Autodesk Fusion 360 part; units mm, degrees
(part 2 of 14)
  arc A256 (88.9, 8.89) -> (88.9, 3.81) centre (88.9, 6.35) ccw
  line L628 (88.646, 6.35) -> (89.154, 6.35)
  line L629 (88.646, 6.35) -> (89.154, 6.35)
  line L630 (88.646, 6.35) -> (89.154, 6.35)
  arc A257 (88.9, 7.62) -> (88.9, 5.08) centre (88.9, 6.35) ccw
  arc A258 (89.5414, 57.15) -> (88.2587, 57.15) centre (88.9, 57.15) ccw
  arc A259 (89.5414, 6.35) -> (88.2587, 6.35) centre (88.9, 6.35) ccw
  line L631 (88.9, 56.896) -> (88.9, 57.404)
  arc A260 (88.9, 5.08) -> (88.9, 7.62) centre (88.9, 6.35) ccw
  arc A261 (89.5414, 6.35) -> (88.2587, 6.35) centre (88.9, 6.35) ccw
  arc A262 (89.5414, 57.15) -> (88.2587, 57.15) centre (88.9, 57.15) ccw
  line L632 (88.646, 6.35) -> (89.154, 6.35)
  line L633 (88.9, 6.096) -> (88.9, 6.604)
  arc A263 (92.31, 13.414) -> (92.31, 12.906) centre (92.31, 13.16) ccw
  arc A264 (89.5414, 6.35) -> (88.2587, 6.35) centre (88.9, 6.35) ccw
  arc A265 (89.5414, 57.15) -> (88.2587, 57.15) centre (88.9, 57.15) ccw
  line L634 (88.9, 6.096) -> (88.9, 6.604)
  line L635 (88.9, 6.096) -> (88.9, 6.604)
  line L636 (88.9, 56.896) -> (88.9, 57.404)
  line L637 (88.646, 57.15) -> (89.154, 57.15)
  arc A266 (88.9, 5.08) -> (88.9, 7.62) centre (88.9, 6.35) ccw
  arc A267 (88.9, 7.62) -> (88.9, 5.08) centre (88.9, 6.35) ccw
  arc A268 (88.9, 4.7879) -> (88.9, 7.9121) centre (88.9, 6.35) ccw
  line L638 (88.9, 56.896) -> (88.9, 57.404)
  arc A269 (89.5414, 57.15) -> (88.2587, 57.15) centre (88.9, 57.15) ccw
  line L639 (88.646, 6.35) -> (89.154, 6.35)
  arc A270 (88.9, 7.9121) -> (88.9, 4.7879) centre (88.9, 6.35) ccw
  arc A271 (88.2587, 6.35) -> (89.5414, 6.35) centre (88.9, 6.35) ccw
  line L640 (88.9, 56.896) -> (88.9, 57.404)
  arc A272 (88.2587, 6.35) -> (89.5414, 6.35) centre (88.9, 6.35) ccw
  line L641 (88.646, 57.15) -> (89.154, 57.15)
  line L642 (88.646, 6.35) -> (89.154, 6.35)
  line L643 (88.646, 6.35) -> (89.154, 6.35)
  line L644 (88.9, 6.096) -> (88.9, 6.604)
  arc A273 (89.5414, 6.35) -> (88.2587, 6.35) centre (88.9, 6.35) ccw
  arc A274 (88.9, 4.7879) -> (88.9, 7.9121) centre (88.9, 6.35) ccw
  arc A275 (88.9, 7.9121) -> (88.9, 4.7879) centre (88.9, 6.35) ccw
  line L645 (88.646, 6.35) -> (89.154, 6.35)
  arc A276 (87.3252, 6.35) -> (90.4748, 6.35) centre (88.9, 6.35) ccw
  arc A277 (87.3252, 6.35) -> (90.4748, 6.35) centre (88.9, 6.35) ccw
  arc A278 (89.5414, 6.35) -> (88.2587, 6.35) centre (88.9, 6.35) ccw
  arc A279 (89.5414, 6.35) -> (88.2587, 6.35) centre (88.9, 6.35) ccw
  arc A280 (88.9, 3.81) -> (88.9, 8.89) centre (88.9, 6.35) ccw
  arc A281 (92.31, 13.668) -> (92.31, 12.652) centre (92.31, 13.16) ccw
  arc A282 (88.9, 8.89) -> (88.9, 3.81) centre (88.9, 6.35) ccw
  arc A283 (90.4748, 57.15) -> (87.3252, 57.15) centre (88.9, 57.15) ccw
  arc A284 (88.2587, 57.15) -> (89.5414, 57.15) centre (88.9, 57.15) ccw
  line L646 (88.9, 6.096) -> (88.9, 6.604)
  arc A285 (92.31, 12.906) -> (92.31, 13.414) centre (92.31, 13.16) ccw
  arc A286 (88.2587, 6.35) -> (89.5414, 6.35) centre (88.9, 6.35) ccw
  arc A287 (88.9, 8.89) -> (88.9, 3.81) centre (88.9, 6.35) ccw
  arc A288 (90.4748, 6.35) -> (87.3252, 6.35) centre (88.9, 6.35) ccw
  line L647 (88.646, 6.35) -> (89.154, 6.35)
  arc A289 (88.2587, 6.35) -> (89.5414, 6.35) centre (88.9, 6.35) ccw
  line L648 (88.9, 6.096) -> (88.9, 6.604)
  arc A290 (89.5414, 6.35) -> (88.2587, 6.35) centre (88.9, 6.35) ccw
  arc A291 (88.2587, 6.35) -> (89.5414, 6.35) centre (88.9, 6.35) ccw
  arc A292 (88.2587, 57.15) -> (89.5414, 57.15) centre (88.9, 57.15) ccw
  arc A293 (88.9, 58.42) -> (88.9, 55.88) centre (88.9, 57.15) ccw
  line L649 (6.35, 56.896) -> (6.35, 57.404)
  arc A294 (88.9, 58.42) -> (88.9, 55.88) centre (88.9, 57.15) ccw
  arc A295 (6.9913, 57.15) -> (5.7086, 57.15) centre (6.35, 57.15) ccw
  arc A296 (4.7752, 57.15) -> (7.9248, 57.15) centre (6.35, 57.15) ccw
  arc A297 (89.5414, 57.15) -> (88.2587, 57.15) centre (88.9, 57.15) ccw
  line L650 (88.646, 57.15) -> (89.154, 57.15)
  arc A298 (88.9, 5.08) -> (88.9, 7.62) centre (88.9, 6.35) ccw
  arc A299 (88.9, 7.62) -> (88.9, 5.08) centre (88.9, 6.35) ccw
  arc A300 (89.5414, 57.15) -> (88.2587, 57.15) centre (88.9, 57.15) ccw
  arc A301 (88.2587, 57.15) -> (89.5414, 57.15) centre (88.9, 57.15) ccw
  arc A302 (88.9, 6.0007) -> (88.9, 6.6992) centre (88.9, 6.35) ccw
  arc A303 (89.5414, 57.15) -> (88.2587, 57.15) centre (88.9, 57.15) ccw
  line L651 (88.646, 57.15) -> (89.154, 57.15)
  arc A304 (88.9, 54.61) -> (88.9, 59.69) centre (88.9, 57.15) ccw
  arc A305 (88.9, 57.931) -> (88.9, 56.3689) centre (88.9, 57.15) ccw
  arc A306 (6.9913, 57.15) -> (5.7086, 57.15) centre (6.35, 57.15) ccw
  arc A307 (88.9, 54.61) -> (88.9, 59.69) centre (88.9, 57.15) ccw
  arc A308 (88.9, 58.42) -> (88.9, 55.88) centre (88.9, 57.15) ccw
  arc A309 (88.9, 58.7121) -> (88.9, 55.5879) centre (88.9, 57.15) ccw
  arc A310 (5.7086, 57.15) -> (6.9913, 57.15) centre (6.35, 57.15) ccw
  line L652 (88.646, 57.15) -> (89.154, 57.15)
  arc A311 (89.5414, 57.15) -> (88.2587, 57.15) centre (88.9, 57.15) ccw
  arc A312 (88.9, 57.4992) -> (88.9, 56.8007) centre (88.9, 57.15) ccw
  line L653 (6.096, 57.15) -> (6.604, 57.15)
  arc A313 (88.2587, 57.15) -> (89.5414, 57.15) centre (88.9, 57.15) ccw
  arc A314 (5.7086, 57.15) -> (6.9913, 57.15) centre (6.35, 57.15) ccw
  line L654 (6.096, 57.15) -> (6.604, 57.15)
  arc A315 (90.4748, 57.15) -> (87.3252, 57.15) centre (88.9, 57.15) ccw
  arc A316 (88.9, 6.6992) -> (88.9, 6.0007) centre (88.9, 6.35) ccw
  line L655 (88.9, 56.896) -> (88.9, 57.404)
  arc A317 (88.2587, 57.15) -> (89.5414, 57.15) centre (88.9, 57.15) ccw
  arc A318 (88.9, 5.08) -> (88.9, 7.62) centre (88.9, 6.35) ccw
  arc A319 (88.2587, 57.15) -> (89.5414, 57.15) centre (88.9, 57.15) ccw
  line L656 (88.646, 57.15) -> (89.154, 57.15)
  line L657 (88.9, 56.896) -> (88.9, 57.404)
  arc A320 (87.3252, 57.15) -> (90.4748, 57.15) centre (88.9, 57.15) ccw
  arc A321 (89.5414, 57.15) -> (88.2587, 57.15) centre (88.9, 57.15) ccw
  line L658 (88.646, 57.15) -> (89.154, 57.15)
  line L659 (88.9, 56.896) -> (88.9, 57.404)
  arc A322 (88.9, 7.62) -> (88.9, 5.08) centre (88.9, 6.35) ccw
  arc A323 (87.3252, 57.15) -> (90.4748, 57.15) centre (88.9, 57.15) ccw
  arc A324 (88.2587, 57.15) -> (89.5414, 57.15) centre (88.9, 57.15) ccw
  arc A325 (88.9, 8.89) -> (88.9, 3.81) centre (88.9, 6.35) ccw
  arc A326 (88.9, 59.69) -> (88.9, 54.61) centre (88.9, 57.15) ccw
  line L660 (88.646, 57.15) -> (89.154, 57.15)
  line L661 (88.9, 56.896) -> (88.9, 57.404)
  arc A327 (88.9, 3.81) -> (88.9, 8.89) centre (88.9, 6.35) ccw
  line L662 (88.646, 57.15) -> (89.154, 57.15)
  arc A328 (88.2587, 57.15) -> (89.5414, 57.15) centre (88.9, 57.15) ccw
  arc A329 (6.9913, 57.15) -> (5.7086, 57.15) centre (6.35, 57.15) ccw
  arc A330 (6.9913, 57.15) -> (5.7086, 57.15) centre (6.35, 57.15) ccw
  arc A331 (88.9, 59.69) -> (88.9, 54.61) centre (88.9, 57.15) ccw
  arc A332 (88.9, 58.7121) -> (88.9, 55.5879) centre (88.9, 57.15) ccw
  arc A333 (88.9, 58.42) -> (88.9, 55.88) centre (88.9, 57.15) ccw
  arc A334 (88.9, 55.88) -> (88.9, 58.42) centre (88.9, 57.15) ccw
  arc A335 (88.9, 55.88) -> (88.9, 58.42) centre (88.9, 57.15) ccw
  arc A336 (4.7752, 57.15) -> (7.9248, 57.15) centre (6.35, 57.15) ccw
  arc A337 (88.9, 55.88) -> (88.9, 58.42) centre (88.9, 57.15) ccw
  line L663 (6.35, 56.896) -> (6.35, 57.404)
  line L664 (21.5392, 25.527) -> (22.1488, 25.527)
  arc A338 (23.16, 24.4688) -> (23.16, 24.4692) centre (23.16, 24.469) ccw
  arc A339 (21.544, 25.5688) -> (21.544, 25.5692) centre (21.544, 25.569) ccw
  line L665 (23.16, 25.569) -> (22.56, 25.569)
  arc A340 (22.144, 25.5688) -> (22.144, 25.5692) centre (22.144, 25.569) ccw
  line L666 (22.5552, 24.894) -> (23.1648, 24.894)
  line L667 (21.5392, 24.511) -> (21.5392, 25.527)
  arc A341 (22.56, 25.5688) -> (22.56, 25.5692) centre (22.56, 25.569) ccw
  line L668 (22.1488, 25.527) -> (22.1488, 24.511)
  line L669 (68.836, 31.9532) -> (69.086, 31.9532)
  line L670 (69.469, 32.5628) -> (69.469, 31.9532)
  arc A342 (21.544, 24.4688) -> (21.544, 24.4692) centre (21.544, 24.469) ccw
  line L671 (22.1488, 25.144) -> (21.5392, 25.144)
  line L672 (68.453, 31.9532) -> (68.453, 32.5628)
  line L673 (22.144, 24.469) -> (22.144, 25.569)
  line L674 (22.56, 24.469) -> (23.16, 24.469)
  arc A343 (23.16, 25.5688) -> (23.16, 25.5692) centre (23.16, 25.569) ccw
  arc A344 (22.56, 25.5692) -> (22.56, 25.5688) centre (22.56, 25.569) ccw
  line L675 (22.56, 25.569) -> (22.56, 24.469)
  line L676 (68.453, 32.5628) -> (69.469, 32.5628)
  line L677 (69.469, 32.5628) -> (69.469, 31.9532)
  line L678 (68.453, 31.9532) -> (68.453, 32.5628)
  arc A345 (21.544, 24.4692) -> (21.544, 24.4688) centre (21.544, 24.469) ccw
  line L679 (21.5392, 25.144) -> (21.5392, 24.894)
  arc A346 (23.16, 24.4692) -> (23.16, 24.4688) centre (23.16, 24.469) ccw
  arc A347 (22.144, 25.5692) -> (22.144, 25.5688) centre (22.144, 25.569) ccw
  line L680 (4.3028, 23.1572) -> (4.9124, 23.1572)
  arc A348 (4.9076, 22.0989) -> (4.9076, 22.0994) centre (4.9076, 22.0992) ccw
  line L681 (23.1648, 25.527) -> (23.1648, 24.511)
  line L682 (4.3076, 22.0992) -> (4.9076, 22.0992)
  line L683 (4.9124, 23.1572) -> (4.9124, 22.1412)
  line L684 (23.1648, 24.511) -> (22.5552, 24.511)
  line L685 (23.1648, 24.511) -> (22.5552, 24.511)
  line L686 (4.3028, 22.5242) -> (4.9124, 22.5242)
  line L687 (4.9076, 23.1992) -> (4.3076, 23.1992)
  line L688 (16.4412, 14.992) -> (15.0188, 14.992)
  arc A349 (4.3076, 23.1989) -> (4.3076, 23.1994) centre (4.3076, 23.1992) ccw
  line L689 (69.469, 31.9532) -> (68.453, 31.9532)
  line L690 (15.0188, 12.706) -> (16.4412, 12.706)
  line L691 (4.3028, 22.1412) -> (4.3028, 23.1572)
  line L692 (22.5552, 25.144) -> (22.5552, 24.894)
  line L693 (68.453, 32.5628) -> (69.469, 32.5628)
  arc A350 (4.9076, 22.0994) -> (4.9076, 22.0989) centre (4.9076, 22.0992) ccw
  line L694 (4.9124, 22.1412) -> (4.3028, 22.1412)
  line L695 (23.1648, 25.527) -> (23.1648, 24.511)
  line L696 (22.5552, 25.527) -> (23.1648, 25.527)
  line L697 (23.1648, 25.144) -> (22.5552, 25.144)
  line L698 (22.5552, 25.527) -> (23.1648, 25.527)
  line L699 (4.3028, 22.7741) -> (4.3028, 22.5242)
  line L700 (4.3028, 22.1412) -> (4.3028, 23.1572)
  arc A351 (16.455, 12.7488) -> (16.455, 12.7493) centre (16.455, 12.749) ccw
  line L701 (16.455, 14.949) -> (15.005, 14.949)
  line L702 (22.5552, 24.511) -> (22.5552, 25.527)
  arc A352 (16.455, 12.7493) -> (16.455, 12.7488) centre (16.455, 12.749) ccw
  line L703 (23.1648, 24.894) -> (23.1648, 25.144)
  line L704 (4.3076, 23.1992) -> (4.3076, 22.0992)
  line L705 (16.455, 12.749) -> (16.455, 14.949)
  line L706 (4.9124, 22.1412) -> (4.3028, 22.1412)
  line L707 (22.5552, 24.511) -> (22.5552, 25.527)
  line L708 (4.9124, 22.5242) -> (4.9124, 22.7741)
  line L709 (4.9124, 22.7741) -> (4.3028, 22.7741)
  arc A353 (4.3076, 22.0989) -> (4.3076, 22.0994) centre (4.3076, 22.0992) ccw
  line L710 (68.58, 22.35) -> (68.58, 22.7)
  line L711 (68.58, 22.35) -> (68.58, 22.7)
  line L712 (4.9076, 22.0992) -> (4.9076, 23.1992)
  line L713 (16.4412, 12.706) -> (16.4412, 14.992)
  line L714 (68.745, 22.54) -> (68.415, 22.54)
  arc A354 (4.3076, 23.1994) -> (4.3076, 23.1989) centre (4.3076, 23.1992) ccw
  line L715 (16.405, 14.699) -> (15.055, 14.699)
  arc A355 (15.005, 14.9492) -> (15.005, 14.9488) centre (15.005, 14.949) ccw
  arc A356 (4.3076, 22.0994) -> (4.3076, 22.0989) centre (4.3076, 22.0992) ccw
  line L716 (16.405, 14.699) -> (15.055, 14.699)
  arc A357 (15.005, 14.9488) -> (15.005, 14.9492) centre (15.005, 14.949) ccw
  arc A358 (4.9076, 23.1994) -> (4.9076, 23.1989) centre (4.9076, 23.1992) ccw
  line L717 (16.4412, 14.992) -> (15.0188, 14.992)
  line L718 (15.0188, 12.706) -> (16.4412, 12.706)
  line L719 (68.58, 22.35) -> (68.58, 22.7)
  arc A359 (82.781, 27.1767) -> (82.781, 27.1132) centre (82.781, 27.145) ccw
  arc A360 (83.081, 27.1767) -> (83.081, 27.1132) centre (83.081, 27.145) ccw
  line L720 (68.7578, 22.5552) -> (68.4022, 22.5552)
  line L721 (15.0188, 14.992) -> (15.0188, 12.706)
  arc A361 (16.455, 14.9492) -> (16.455, 14.9488) centre (16.455, 14.949) ccw
  arc A362 (16.455, 14.9488) -> (16.455, 14.9492) centre (16.455, 14.949) ccw
  arc A363 (4.9076, 23.1989) -> (4.9076, 23.1994) centre (4.9076, 23.1992) ccw
  line L722 (15.0188, 14.992) -> (15.0188, 12.706)
  line L723 (15.005, 14.949) -> (15.005, 12.749)
  line L724 (15.005, 12.749) -> (16.455, 12.749)
  line L725 (16.4412, 12.706) -> (16.4412, 14.992)
  line L726 (16.405, 12.999) -> (15.055, 12.999)
  line L727 (4.3028, 23.1572) -> (4.9124, 23.1572)
  line L728 (68.43, 21.75) -> (68.73, 21.75)
  line L729 (68.73, 21.75) -> (68.73, 22.7)
  line L730 (4.9124, 23.1572) -> (4.9124, 22.1412)
  arc A364 (68.43, 22.7317) -> (68.43, 22.6682) centre (68.43, 22.7) ccw
  arc A365 (33.1967, 60.17) -> (33.1972, 60.17) centre (33.197, 60.17) ccw
  arc A366 (33.1967, 58.138) -> (33.1972, 58.138) centre (33.197, 58.138) ccw
  arc A367 (34.2972, 60.17) -> (34.2967, 60.17) centre (34.297, 60.17) ccw
  line L731 (33.872, 58.7428) -> (33.622, 58.7428)
  line L732 (33.622, 58.1332) -> (33.872, 58.1332)
  line L733 (33.622, 58.438) -> (33.072, 58.438)
  arc A368 (34.2967, 58.138) -> (34.2972, 58.138) centre (34.297, 58.138) ccw
  line L734 (34.422, 58.438) -> (33.872, 58.438)
  line L735 (33.239, 58.1332) -> (33.239, 58.7428)
  arc A369 (34.2967, 59.754) -> (34.2972, 59.754) centre (34.297, 59.754) ccw
  line L736 (33.872, 60.7748) -> (33.622, 60.7748)
  line L737 (34.255, 60.1652) -> (33.239, 60.1652)
  line L738 (33.239, 58.7428) -> (34.255, 58.7428)
  line L739 (34.422, 58.438) -> (33.872, 58.438)
  line L740 (34.255, 60.7748) -> (34.255, 60.1652)
  line L741 (33.622, 60.7748) -> (33.622, 60.1652)
  line L742 (34.255, 59.7588) -> (34.255, 59.1492)
  line L743 (34.255, 59.1492) -> (33.239, 59.1492)
  line L744 (34.255, 58.7428) -> (34.255, 58.1332)
  line L745 (33.239, 59.1492) -> (33.239, 59.7588)
  arc A370 (34.2967, 59.154) -> (34.2972, 59.154) centre (34.297, 59.154) ccw
  arc A371 (34.2972, 60.77) -> (34.2967, 60.77) centre (34.297, 60.77) ccw
  line L746 (33.239, 59.7588) -> (34.255, 59.7588)
  line L747 (33.622, 60.1652) -> (33.872, 60.1652)
  line L748 (34.255, 59.1492) -> (33.239, 59.1492)
  arc A372 (33.1967, 59.154) -> (33.1972, 59.154) centre (33.197, 59.154) ccw
  arc A373 (34.2967, 60.77) -> (34.2972, 60.77) centre (34.297, 60.77) ccw
  arc A374 (33.1972, 59.154) -> (33.1967, 59.154) centre (33.197, 59.154) ccw
  line L749 (33.239, 60.7748) -> (34.255, 60.7748)
  arc A375 (33.1972, 59.754) -> (33.1967, 59.754) centre (33.197, 59.754) ccw
  line L750 (33.239, 59.7588) -> (34.255, 59.7588)
  line L751 (34.255, 60.1652) -> (33.239, 60.1652)
  line L752 (34.422, 59.454) -> (33.872, 59.454)
  line L753 (33.622, 59.7588) -> (33.622, 59.1492)
  line L754 (34.422, 59.454) -> (33.872, 59.454)
  line L755 (34.255, 59.7588) -> (34.255, 59.1492)
  arc A376 (33.1967, 59.754) -> (33.1972, 59.754) centre (33.197, 59.754) ccw
  line L756 (33.872, 59.7588) -> (33.622, 59.7588)
  arc A377 (34.2972, 59.154) -> (34.2967, 59.154) centre (34.297, 59.154) ccw
  line L757 (33.622, 59.454) -> (33.072, 59.454)
  line L758 (34.297, 60.17) -> (34.297, 60.77)
  line L759 (33.622, 59.454) -> (33.072, 59.454)
  arc A378 (34.2972, 59.754) -> (34.2967, 59.754) centre (34.297, 59.754) ccw
  line L760 (33.197, 60.17) -> (34.297, 60.17)
  line L761 (33.239, 60.1652) -> (33.239, 60.7748)
  arc A379 (33.1972, 60.77) -> (33.1967, 60.77) centre (33.197, 60.77) ccw
  line L762 (33.872, 60.1652) -> (33.872, 60.7748)
  arc A380 (34.2967, 60.17) -> (34.2972, 60.17) centre (34.297, 60.17) ccw
  line L763 (34.255, 60.7748) -> (34.255, 60.1652)
  line L764 (34.297, 60.77) -> (33.197, 60.77)
  line L765 (34.422, 59.454) -> (33.872, 59.454)
  line L766 (33.239, 60.1652) -> (33.239, 60.7748)
  line L767 (33.197, 60.77) -> (33.197, 60.17)
  line L768 (33.239, 60.7748) -> (34.255, 60.7748)
  arc A381 (33.1972, 60.17) -> (33.1967, 60.17) centre (33.197, 60.17) ccw
  line L769 (33.239, 59.1492) -> (33.239, 59.7588)
  line L770 (33.622, 59.1492) -> (33.872, 59.1492)
  arc A382 (33.1967, 60.77) -> (33.1972, 60.77) centre (33.197, 60.77) ccw
  line L771 (33.239, 61.7908) -> (34.255, 61.7908)
  arc A383 (34.2967, 61.186) -> (34.2972, 61.186) centre (34.297, 61.186) ccw
  line L772 (34.422, 61.486) -> (33.872, 61.486)
  line L773 (33.197, 61.186) -> (34.297, 61.186)
  line L774 (34.255, 61.1812) -> (33.239, 61.1812)
  line L775 (33.622, 59.454) -> (33.072, 59.454)
  line L776 (33.872, 61.1812) -> (33.872, 61.7908)
  line L777 (33.622, 61.1812) -> (33.872, 61.1812)
  line L778 (33.622, 60.47) -> (33.072, 60.47)
  arc A384 (34.2967, 61.786) -> (34.2972, 61.786) centre (34.297, 61.786) ccw
  line L779 (33.622, 60.47) -> (33.072, 60.47)
  line L780 (34.422, 61.486) -> (33.872, 61.486)
  line L781 (34.422, 60.47) -> (33.872, 60.47)
  line L782 (33.239, 61.1812) -> (33.239, 61.7908)
  line L783 (34.297, 61.186) -> (34.297, 61.786)
  arc A385 (33.1967, 61.786) -> (33.1972, 61.786) centre (33.197, 61.786) ccw
  line L784 (33.622, 61.7908) -> (33.622, 61.1812)
  line L785 (34.255, 61.7908) -> (34.255, 61.1812)
  line L786 (34.297, 61.786) -> (33.197, 61.786)
  arc A386 (33.1972, 61.186) -> (33.1967, 61.186) centre (33.197, 61.186) ccw
  arc A387 (33.1972, 61.786) -> (33.1967, 61.786) centre (33.197, 61.786) ccw
  line L787 (34.422, 60.47) -> (33.872, 60.47)
  line L788 (34.255, 61.1812) -> (33.239, 61.1812)
  line L789 (34.255, 61.7908) -> (34.255, 61.1812)
  line L790 (33.197, 61.786) -> (33.197, 61.186)
  line L791 (33.239, 61.1812) -> (33.239, 61.7908)
  arc A388 (33.1967, 61.186) -> (33.1972, 61.186) centre (33.197, 61.186) ccw
  arc A389 (34.2972, 61.786) -> (34.2967, 61.786) centre (34.297, 61.786) ccw
  line L792 (34.422, 60.47) -> (33.872, 60.47)
  line L793 (30.311, 59.228) -> (30.311, 58.628)
  line L794 (30.736, 58.6232) -> (30.986, 58.6232)
  line L795 (33.622, 61.486) -> (33.072, 61.486)
  line L796 (33.622, 60.47) -> (33.072, 60.47)
  arc A390 (34.2972, 61.186) -> (34.2967, 61.186) centre (34.297, 61.186) ccw
  line L797 (30.311, 58.628) -> (31.411, 58.628)
  line L798 (33.872, 61.7908) -> (33.622, 61.7908)
  arc A391 (31.4112, 58.628) -> (31.4108, 58.628) centre (31.411, 58.628) ccw
  line L799 (33.622, 61.486) -> (33.072, 61.486)
  line L800 (30.353, 58.6232) -> (30.353, 59.2328)
  line L801 (33.622, 61.486) -> (33.072, 61.486)
  line L802 (33.239, 61.7908) -> (34.255, 61.7908)
  line L803 (31.411, 59.228) -> (30.311, 59.228)
  line L804 (30.311, 57.612) -> (31.411, 57.612)
  line L805 (34.422, 61.486) -> (33.872, 61.486)
  line L806 (31.411, 57.612) -> (31.411, 58.212)
  line L807 (31.411, 58.212) -> (30.311, 58.212)
  line L808 (31.369, 59.2328) -> (31.369, 58.6232)
  line L809 (30.986, 58.928) -> (31.536, 58.928)
  line L810 (30.311, 58.212) -> (30.311, 57.612)
  arc A392 (31.4108, 59.228) -> (31.4112, 59.228) centre (31.411, 59.228) ccw
  arc A393 (31.4112, 57.612) -> (31.4108, 57.612) centre (31.411, 57.612) ccw
  line L811 (30.186, 58.928) -> (30.736, 58.928)
  line L812 (30.186, 58.928) -> (30.736, 58.928)
  line L813 (30.353, 58.2168) -> (31.369, 58.2168)
  line L814 (30.353, 59.2328) -> (31.369, 59.2328)
  arc A394 (31.4108, 57.612) -> (31.4112, 57.612) centre (31.411, 57.612) ccw
  arc A395 (31.4108, 58.212) -> (31.4112, 58.212) centre (31.411, 58.212) ccw
  arc A396 (30.3112, 59.228) -> (30.3108, 59.228) centre (30.311, 59.228) ccw
  line L815 (31.369, 58.6232) -> (30.353, 58.6232)
  arc A397 (30.3112, 57.612) -> (30.3108, 57.612) centre (30.311, 57.612) ccw
  line L816 (31.369, 57.6072) -> (30.353, 57.6072)
  line L817 (30.353, 57.6072) -> (30.353, 58.2168)
  line L818 (30.736, 59.2328) -> (30.736, 58.6232)
  arc A398 (31.4108, 58.628) -> (31.4112, 58.628) centre (31.411, 58.628) ccw
  line L819 (30.186, 58.928) -> (30.736, 58.928)
  line L820 (30.353, 58.6232) -> (30.353, 59.2328)
  arc A399 (30.3112, 58.628) -> (30.3108, 58.628) centre (30.311, 58.628) ccw
  arc A400 (30.3108, 57.612) -> (30.3112, 57.612) centre (30.311, 57.612) ccw
  line L821 (30.986, 58.928) -> (31.536, 58.928)
  line L822 (31.369, 58.2168) -> (31.369, 57.6072)
  arc A401 (30.3108, 58.628) -> (30.3112, 58.628) centre (30.311, 58.628) ccw
  line L823 (31.369, 58.6232) -> (30.353, 58.6232)
  arc A402 (31.4112, 58.212) -> (31.4108, 58.212) centre (31.411, 58.212) ccw
  arc A403 (30.3108, 58.212) -> (30.3112, 58.212) centre (30.311, 58.212) ccw
  arc A404 (30.3112, 58.212) -> (30.3108, 58.212) centre (30.311, 58.212) ccw
  line L824 (30.736, 58.2168) -> (30.736, 57.6072)
  arc A405 (31.4112, 59.228) -> (31.4108, 59.228) centre (31.411, 59.228) ccw
  line L825 (31.411, 58.628) -> (31.411, 59.228)
  line L826 (31.369, 59.2328) -> (31.369, 58.6232)
  line L827 (30.986, 59.2328) -> (30.736, 59.2328)
  line L828 (30.986, 58.6232) -> (30.986, 59.2328)
  line L829 (29.7688, 50.165) -> (29.1592, 50.165)
  line L830 (30.186, 57.912) -> (30.736, 57.912)
  line L831 (30.186, 57.912) -> (30.736, 57.912)
  line L832 (30.986, 57.6072) -> (30.986, 58.2168)
  line L833 (29.464, 51.348) -> (29.464, 50.798)
  arc A406 (29.164, 51.2232) -> (29.164, 51.2228) centre (29.164, 51.223) ccw
  line L834 (29.7688, 51.181) -> (29.7688, 50.165)
  line L835 (29.164, 50.123) -> (29.764, 50.123)
  line L836 (30.986, 57.912) -> (31.536, 57.912)
  arc A407 (29.764, 50.1232) -> (29.764, 50.1228) centre (29.764, 50.123) ccw
  arc A408 (29.164, 50.1232) -> (29.164, 50.1228) centre (29.164, 50.123) ccw
  line L837 (30.986, 57.912) -> (31.536, 57.912)
  line L838 (29.1592, 50.548) -> (29.7688, 50.548)
  arc A409 (29.764, 51.2228) -> (29.764, 51.2232) centre (29.764, 51.223) ccw
  line L839 (30.986, 58.928) -> (31.536, 58.928)
  line L840 (29.1592, 50.798) -> (29.1592, 50.548)
  line L841 (29.1592, 51.181) -> (29.7688, 51.181)
  arc A410 (30.3108, 59.228) -> (30.3112, 59.228) centre (30.311, 59.228) ccw
  line L842 (31.369, 58.2168) -> (31.369, 57.6072)
  line L843 (31.369, 57.6072) -> (30.353, 57.6072)
  line L844 (30.986, 57.912) -> (31.536, 57.912)
  arc A411 (29.164, 50.1228) -> (29.164, 50.1232) centre (29.164, 50.123) ccw
  line L845 (30.353, 57.6072) -> (30.353, 58.2168)
  line L846 (29.7688, 51.181) -> (29.7688, 50.165)
  line L847 (29.164, 51.223) -> (29.164, 50.123)
  arc A412 (29.764, 50.1228) -> (29.764, 50.1232) centre (29.764, 50.123) ccw
  line L848 (29.464, 51.348) -> (29.464, 50.798)
  line L849 (29.764, 51.223) -> (29.164, 51.223)
  arc A413 (29.164, 51.2228) -> (29.164, 51.2232) centre (29.164, 51.223) ccw
  line L850 (30.353, 59.2328) -> (31.369, 59.2328)
  line L851 (30.186, 57.912) -> (30.736, 57.912)
  line L852 (29.1592, 50.165) -> (29.1592, 51.181)
  line L853 (29.1592, 50.165) -> (29.1592, 51.181)
  line L854 (29.7688, 50.548) -> (29.7688, 50.798)
  arc A414 (29.764, 51.2232) -> (29.764, 51.2228) centre (29.764, 51.223) ccw
  line L855 (29.1592, 51.181) -> (29.7688, 51.181)
  line L856 (30.736, 57.6072) -> (30.986, 57.6072)
  line L857 (29.7688, 50.798) -> (29.1592, 50.798)
  line L858 (29.7688, 50.165) -> (29.1592, 50.165)
  line L859 (29.464, 51.348) -> (29.464, 50.798)
  line L860 (30.353, 58.2168) -> (31.369, 58.2168)
  line L861 (29.764, 50.123) -> (29.764, 51.223)
  arc A415 (75.357, 33.3588) -> (75.357, 33.3592) centre (75.357, 33.359) ccw
  line L862 (75.3618, 34.034) -> (74.7522, 34.034)
  line L863 (75.3618, 33.401) -> (74.7522, 33.401)
  line L864 (30.986, 58.2168) -> (30.736, 58.2168)
  line L865 (75.357, 33.359) -> (75.357, 34.459)
  line L866 (75.357, 34.459) -> (74.757, 34.459)
  line L867 (74.7522, 33.401) -> (74.7522, 34.417)
  arc A416 (74.757, 34.4592) -> (74.757, 34.4588) centre (74.757, 34.459) ccw
  arc A417 (74.757, 33.3588) -> (74.757, 33.3592) centre (74.757, 33.359) ccw
  line L868 (74.7522, 34.417) -> (75.3618, 34.417)
  line L869 (75.3618, 34.417) -> (75.3618, 33.401)
  arc A418 (77.043, 54.9058) -> (77.043, 54.9062) centre (77.043, 54.906) ccw
  line L870 (75.057, 34.034) -> (75.057, 34.584)
  arc A419 (74.757, 34.4588) -> (74.757, 34.4592) centre (74.757, 34.459) ccw
  line L871 (75.3618, 33.784) -> (75.3618, 34.034)
  line L872 (77.043, 53.806) -> (77.643, 53.806)
  arc A420 (77.643, 53.8058) -> (77.643, 53.8062) centre (77.643, 53.806) ccw
  line L873 (77.043, 54.906) -> (77.043, 53.806)
  line L874 (29.464, 50.548) -> (29.464, 49.998)
  arc A421 (77.643, 53.8062) -> (77.643, 53.8058) centre (77.643, 53.806) ccw
  arc A422 (77.643, 54.9058) -> (77.643, 54.9062) centre (77.643, 54.906) ccw
  arc A423 (75.357, 34.4592) -> (75.357, 34.4588) centre (75.357, 34.459) ccw
  line L875 (77.0382, 54.231) -> (77.6478, 54.231)
  arc A424 (74.757, 33.3592) -> (74.757, 33.3588) centre (74.757, 33.359) ccw
  arc A425 (77.643, 54.9062) -> (77.643, 54.9058) centre (77.643, 54.906) ccw
  line L876 (74.757, 33.359) -> (75.357, 33.359)
  line L877 (77.643, 54.906) -> (77.043, 54.906)
  line L878 (75.057, 33.234) -> (75.057, 33.784)
  line L879 (74.757, 34.459) -> (74.757, 33.359)
  line L880 (74.7522, 34.417) -> (75.3618, 34.417)
  line L881 (75.3618, 34.417) -> (75.3618, 33.401)
  line L882 (75.057, 33.234) -> (75.057, 33.784)
  line L883 (34.802, 40.8552) -> (34.802, 41.4648)
  arc A426 (34.7602, 40.86) -> (34.7598, 40.86) centre (34.76, 40.86) ccw
  arc A427 (35.8597, 41.46) -> (35.8602, 41.46) centre (35.86, 41.46) ccw
  line L884 (29.464, 50.548) -> (29.464, 49.998)
  arc A428 (77.043, 53.8062) -> (77.043, 53.8058) centre (77.043, 53.806) ccw
  line L885 (34.76, 40.86) -> (35.86, 40.86)
  line L886 (77.643, 53.806) -> (77.643, 54.906)
  line L887 (75.057, 34.034) -> (75.057, 34.584)
  line L888 (77.0382, 53.848) -> (77.0382, 54.864)
  line L889 (74.7522, 34.034) -> (74.7522, 33.784)
  line L890 (77.6478, 53.848) -> (77.0382, 53.848)
  line L891 (77.6478, 54.231) -> (77.6478, 54.481)
  arc A429 (77.043, 53.8058) -> (77.043, 53.8062) centre (77.043, 53.806) ccw
  arc A430 (34.7598, 41.46) -> (34.7602, 41.46) centre (34.76, 41.46) ccw
  arc A431 (35.8602, 41.46) -> (35.8597, 41.46) centre (35.86, 41.46) ccw
  arc A432 (75.357, 33.3592) -> (75.357, 33.3588) centre (75.357, 33.359) ccw
  line L892 (75.3618, 33.401) -> (74.7522, 33.401)
  line L893 (74.7522, 33.401) -> (74.7522, 34.417)
  arc A433 (75.357, 34.4588) -> (75.357, 34.4592) centre (75.357, 34.459) ccw
  line L894 (77.0382, 54.864) -> (77.6478, 54.864)
  line L895 (77.0382, 54.481) -> (77.0382, 54.231)
  line L896 (74.7522, 33.784) -> (75.3618, 33.784)
  line L897 (75.057, 33.234) -> (75.057, 33.784)
  line L898 (75.057, 34.034) -> (75.057, 34.584)
  line L899 (29.464, 50.548) -> (29.464, 49.998)
  line L900 (77.343, 54.481) -> (77.343, 55.031)
  line L901 (77.6478, 53.848) -> (77.0382, 53.848)
  line L902 (35.818, 41.4648) -> (35.818, 40.8552)
  line L903 (77.343, 54.481) -> (77.343, 55.031)
  arc A434 (34.7598, 40.86) -> (34.7602, 40.86) centre (34.76, 40.86) ccw
  line L904 (34.802, 41.4648) -> (35.818, 41.4648)
  line L905 (34.802, 40.8552) -> (34.802, 41.4648)
  line L906 (77.4192, 33.401) -> (77.4192, 34.417)
  line L907 (77.724, 33.234) -> (77.724, 33.784)
  line L908 (77.724, 34.034) -> (77.724, 34.584)
  line L909 (35.985, 41.16) -> (35.435, 41.16)
  line L910 (77.724, 34.034) -> (77.724, 34.584)
  line L911 (78.024, 34.459) -> (77.424, 34.459)
  arc A435 (77.424, 34.4588) -> (77.424, 34.4592) centre (77.424, 34.459) ccw
  line L912 (35.185, 41.16) -> (34.635, 41.16)
  arc A436 (77.424, 34.4592) -> (77.424, 34.4588) centre (77.424, 34.459) ccw
  line L913 (77.6478, 54.864) -> (77.6478, 53.848)
  line L914 (77.343, 53.681) -> (77.343, 54.231)
  line L915 (78.0288, 34.417) -> (78.0288, 33.401)
  arc A437 (34.7602, 41.46) -> (34.7598, 41.46) centre (34.76, 41.46) ccw
  arc A438 (77.043, 54.9062) -> (77.043, 54.9058) centre (77.043, 54.906) ccw
  line L916 (77.0382, 54.864) -> (77.6478, 54.864)
  line L917 (34.76, 41.46) -> (34.76, 40.86)
  arc A439 (35.8602, 40.86) -> (35.8597, 40.86) centre (35.86, 40.86) ccw
  line L918 (77.6478, 54.864) -> (77.6478, 53.848)
  line L919 (35.185, 40.8552) -> (35.435, 40.8552)
  line L920 (77.6478, 54.481) -> (77.0382, 54.481)
  arc A440 (78.024, 33.3592) -> (78.024, 33.3588) centre (78.024, 33.359) ccw
  line L921 (77.4192, 33.784) -> (78.0288, 33.784)
  line L922 (77.0382, 53.848) -> (77.0382, 54.864)
  line L923 (35.985, 41.16) -> (35.435, 41.16)
  line L924 (35.185, 41.4648) -> (35.185, 40.8552)
  line L925 (77.4192, 33.401) -> (77.4192, 34.417)
  line L926 (35.86, 40.86) -> (35.86, 41.46)
  line L927 (78.024, 33.359) -> (78.024, 34.459)
  arc A441 (78.024, 34.4592) -> (78.024, 34.4588) centre (78.024, 34.459) ccw
  line L928 (78.0288, 33.784) -> (78.0288, 34.034)
  line L929 (34.802, 41.4648) -> (35.818, 41.4648)
  line L930 (35.435, 40.8552) -> (35.435, 41.4648)
  arc A442 (35.8597, 40.86) -> (35.8602, 40.86) centre (35.86, 40.86) ccw
  line L931 (35.818, 41.4648) -> (35.818, 40.8552)
  arc A443 (78.024, 34.4588) -> (78.024, 34.4592) centre (78.024, 34.459) ccw
  line L932 (78.0288, 33.401) -> (77.4192, 33.401)
  line L933 (77.4192, 34.034) -> (77.4192, 33.784)
  line L934 (77.343, 53.681) -> (77.343, 54.231)
  line L935 (35.86, 41.46) -> (34.76, 41.46)
  line L936 (35.818, 40.8552) -> (34.802, 40.8552)
  line L937 (35.435, 41.4648) -> (35.185, 41.4648)
  line L938 (35.185, 41.16) -> (34.635, 41.16)
  line L939 (77.343, 53.681) -> (77.343, 54.231)
  line L940 (35.818, 40.8552) -> (34.802, 40.8552)
  line L941 (77.343, 54.481) -> (77.343, 55.031)
  line L942 (78.0288, 33.401) -> (77.4192, 33.401)
  line L943 (93.458, 38.255) -> (93.458, 39.215)
  line L944 (35.185, 41.16) -> (34.635, 41.16)
  line L945 (73.025, 33.0962) -> (73.025, 33.7058)
  line L946 (91.7448, 38.2524) -> (93.4212, 38.2524)
  line L947 (74.083, 33.701) -> (72.983, 33.701)
  arc A444 (91.7082, 39.215) -> (91.7078, 39.215) centre (91.708, 39.215) ccw
  line L948 (73.658, 33.0962) -> (73.658, 33.7058)
  line L949 (91.7448, 39.2176) -> (91.7448, 38.2524)
  line L950 (74.083, 33.101) -> (74.083, 33.701)
  arc A445 (72.9832, 33.101) -> (72.9828, 33.101) centre (72.983, 33.101) ccw
  arc A446 (72.9828, 33.101) -> (72.9832, 33.101) centre (72.983, 33.101) ccw
  line L951 (73.408, 33.7058) -> (73.408, 33.0962)
  line L952 (77.724, 33.234) -> (77.724, 33.784)
  line L953 (35.985, 41.16) -> (35.435, 41.16)
  line L954 (77.424, 34.459) -> (77.424, 33.359)
  arc A447 (77.424, 33.3588) -> (77.424, 33.3592) centre (77.424, 33.359) ccw
  arc A448 (77.424, 33.3592) -> (77.424, 33.3588) centre (77.424, 33.359) ccw
  line L955 (73.408, 33.0962) -> (73.658, 33.0962)
  arc A449 (74.0832, 33.701) -> (74.0828, 33.701) centre (74.083, 33.701) ccw
  arc A450 (72.9832, 33.701) -> (72.9828, 33.701) centre (72.983, 33.701) ccw
  arc A451 (72.9828, 33.701) -> (72.9832, 33.701) centre (72.983, 33.701) ccw
  line L956 (93.4212, 39.2176) -> (91.7448, 39.2176)
  line L957 (77.424, 33.359) -> (78.024, 33.359)
  arc A452 (74.0828, 33.701) -> (74.0832, 33.701) centre (74.083, 33.701) ccw
  line L958 (91.7448, 39.2176) -> (91.7448, 38.2524)
  line L959 (72.983, 33.701) -> (72.983, 33.101)
  line L960 (73.025, 33.7058) -> (74.041, 33.7058)
  line L961 (74.208, 33.401) -> (73.658, 33.401)
  line L962 (73.408, 33.401) -> (72.858, 33.401)
  line L963 (73.025, 33.0962) -> (73.025, 33.7058)
  line L964 (91.7448, 38.2524) -> (93.4212, 38.2524)
  line L965 (78.0288, 34.417) -> (78.0288, 33.401)
  line L966 (77.724, 34.034) -> (77.724, 34.584)
  line L967 (77.4192, 34.417) -> (78.0288, 34.417)
  arc A453 (78.024, 33.3588) -> (78.024, 33.3592) centre (78.024, 33.359) ccw
  line L968 (93.4212, 39.2176) -> (91.7448, 39.2176)
  line L969 (91.708, 38.255) -> (93.458, 38.255)
  line L970 (73.025, 33.7058) -> (74.041, 33.7058)
  line L971 (74.041, 33.0962) -> (73.025, 33.0962)
  line L972 (77.4192, 34.417) -> (78.0288, 34.417)
  line L973 (77.724, 33.234) -> (77.724, 33.784)
  line L974 (78.0288, 34.034) -> (77.4192, 34.034)
  arc A454 (91.7078, 39.215) -> (91.7082, 39.215) centre (91.708, 39.215) ccw
  arc A455 (91.8352, 53.495) -> (91.8348, 53.495) centre (91.835, 53.495) ccw
  arc A456 (74.0832, 33.101) -> (74.0828, 33.101) centre (74.083, 33.101) ccw
  line L975 (91.883, 38.285) -> (91.883, 39.185)
  arc A457 (93.4582, 39.215) -> (93.4578, 39.215) centre (93.458, 39.215) ccw
  line L976 (93.5482, 53.4924) -> (93.5482, 54.4576)
  line L977 (92.01, 53.525) -> (92.01, 54.425)
  line L978 (93.41, 53.525) -> (93.41, 54.425)
  line L979 (91.883, 38.285) -> (91.883, 39.185)
  line L980 (91.708, 39.215) -> (91.708, 38.255)
  arc A458 (93.5848, 53.495) -> (93.5852, 53.495) centre (93.585, 53.495) ccw
  arc A459 (91.7078, 38.255) -> (91.7082, 38.255) centre (91.708, 38.255) ccw
  line L981 (93.283, 38.285) -> (93.283, 39.185)
  line L982 (74.208, 33.401) -> (73.658, 33.401)
  line L983 (91.883, 38.285) -> (91.883, 39.185)
  line L984 (91.8718, 54.4576) -> (91.8718, 53.4924)
  line L985 (93.5482, 53.4924) -> (93.5482, 54.4576)
  line L986 (93.585, 53.495) -> (93.585, 54.455)
  line L987 (91.835, 53.495) -> (93.585, 53.495)
  arc A460 (93.5848, 54.455) -> (93.5852, 54.455) centre (93.585, 54.455) ccw
  line L988 (74.041, 33.7058) -> (74.041, 33.0962)
  line L989 (93.283, 38.285) -> (93.283, 39.185)
  line L990 (74.208, 33.401) -> (73.658, 33.401)
  line L991 (93.5482, 54.4576) -> (91.8718, 54.4576)
  line L992 (73.658, 33.7058) -> (73.408, 33.7058)
  arc A461 (93.4578, 38.255) -> (93.4582, 38.255) centre (93.458, 38.255) ccw
  line L993 (93.41, 53.525) -> (93.41, 54.425)
  arc A462 (93.5852, 53.495) -> (93.5848, 53.495) centre (93.585, 53.495) ccw
  line L994 (92.01, 53.525) -> (92.01, 54.425)
  arc A463 (91.7082, 38.255) -> (91.7078, 38.255) centre (91.708, 38.255) ccw
  arc A464 (93.5852, 54.455) -> (93.5848, 54.455) centre (93.585, 54.455) ccw
  line L995 (74.041, 33.7058) -> (74.041, 33.0962)
  line L996 (73.408, 33.401) -> (72.858, 33.401)
  arc A465 (93.4582, 38.255) -> (93.4578, 38.255) centre (93.458, 38.255) ccw
  line L997 (93.458, 39.215) -> (91.708, 39.215)
  line L998 (73.408, 33.401) -> (72.858, 33.401)
  line L999 (93.4212, 38.2524) -> (93.4212, 39.2176)
  line L1000 (93.585, 54.455) -> (91.835, 54.455)
  line L1001 (93.4212, 38.2524) -> (93.4212, 39.2176)
  line L1002 (91.835, 23.523) -> (93.585, 23.523)
  line L1003 (74.041, 33.0962) -> (73.025, 33.0962)
  line L1004 (93.41, 53.525) -> (93.41, 54.425)
  arc A466 (74.0828, 33.101) -> (74.0832, 33.101) centre (74.083, 33.101) ccw
  arc A467 (91.8348, 54.455) -> (91.8352, 54.455) centre (91.835, 54.455) ccw
  line L1005 (91.8718, 53.4924) -> (93.5482, 53.4924)
  line L1006 (72.983, 33.101) -> (74.083, 33.101)
  line L1007 (91.8718, 53.4924) -> (93.5482, 53.4924)
  line L1008 (91.8718, 54.4576) -> (91.8718, 53.4924)
  arc A468 (93.4578, 39.215) -> (93.4582, 39.215) centre (93.458, 39.215) ccw
  line L1009 (91.835, 54.455) -> (91.835, 53.495)
  line L1010 (93.41, 23.553) -> (93.41, 24.453)
  arc A469 (91.8352, 24.483) -> (91.8348, 24.483) centre (91.835, 24.483) ccw
  line L1011 (91.962, 9.68) -> (93.712, 9.68)
  line L1012 (93.5482, 24.4856) -> (91.8718, 24.4856)
  line L1013 (93.5482, 23.5204) -> (93.5482, 24.4856)
  line L1014 (91.9988, 10.6426) -> (91.9988, 9.6774)
  arc A470 (93.5852, 24.483) -> (93.5848, 24.483) centre (93.585, 24.483) ccw
  line L1015 (91.8718, 24.4856) -> (91.8718, 23.5204)
  arc A471 (91.9618, 9.68) -> (91.9622, 9.68) centre (91.962, 9.68) ccw
  line L1016 (92.01, 23.553) -> (92.01, 24.453)
  line L1017 (92.01, 53.525) -> (92.01, 54.425)
  line L1018 (92.01, 23.553) -> (92.01, 24.453)
  line L1019 (93.585, 24.483) -> (91.835, 24.483)
  line L1020 (93.6752, 9.6774) -> (93.6752, 10.6426)
  arc A472 (91.8348, 24.483) -> (91.8352, 24.483) centre (91.835, 24.483) ccw
  arc A473 (93.7122, 9.68) -> (93.7118, 9.68) centre (93.712, 9.68) ccw
  arc A474 (93.5852, 23.523) -> (93.5848, 23.523) centre (93.585, 23.523) ccw
  line L1021 (91.9988, 10.6426) -> (91.9988, 9.6774)
  line L1022 (93.6752, 9.6774) -> (93.6752, 10.6426)
  line L1023 (92.137, 9.71) -> (92.137, 10.61)
  arc A475 (91.9622, 9.68) -> (91.9618, 9.68) centre (91.962, 9.68) ccw
  arc A476 (93.5848, 24.483) -> (93.5852, 24.483) centre (93.585, 24.483) ccw
  line L1024 (91.9988, 9.6774) -> (93.6752, 9.6774)
  arc A477 (93.7118, 10.64) -> (93.7122, 10.64) centre (93.712, 10.64) ccw
  arc A478 (91.8352, 54.455) -> (91.8348, 54.455) centre (91.835, 54.455) ccw
  line L1025 (93.6752, 10.6426) -> (91.9988, 10.6426)
  line L1026 (93.41, 23.553) -> (93.41, 24.453)
  line L1027 (93.585, 23.523) -> (93.585, 24.483)
  line L1028 (93.6752, 10.6426) -> (91.9988, 10.6426)
  line L1029 (93.283, 38.285) -> (93.283, 39.185)
  arc A479 (91.8352, 23.523) -> (91.8348, 23.523) centre (91.835, 23.523) ccw
  arc A480 (93.5848, 23.523) -> (93.5852, 23.523) centre (93.585, 23.523) ccw
  arc A481 (91.9618, 10.64) -> (91.9622, 10.64) centre (91.962, 10.64) ccw
  line L1030 (93.5482, 54.4576) -> (91.8718, 54.4576)
  line L1031 (91.962, 10.64) -> (91.962, 9.68)
  line L1032 (93.5482, 24.4856) -> (91.8718, 24.4856)
  arc A482 (91.9622, 10.64) -> (91.9618, 10.64) centre (91.962, 10.64) ccw
  line L1033 (92.01, 23.553) -> (92.01, 24.453)
  line L1034 (91.835, 24.483) -> (91.835, 23.523)
  arc A483 (91.8348, 53.495) -> (91.8352, 53.495) centre (91.835, 53.495) ccw
  line L1035 (93.712, 10.64) -> (91.962, 10.64)
  line L1036 (93.712, 9.68) -> (93.712, 10.64)
  line L1037 (91.8718, 23.5204) -> (93.5482, 23.5204)
  line L1038 (91.8718, 24.4856) -> (91.8718, 23.5204)
  line L1039 (93.41, 23.553) -> (93.41, 24.453)
  line L1040 (91.9988, 9.6774) -> (93.6752, 9.6774)
  arc A484 (93.7118, 9.68) -> (93.7122, 9.68) centre (93.712, 9.68) ccw
  line L1041 (4.8683, 10.2023) -> (4.6887, 10.0227)
  line L1042 (74.208, 36.068) -> (73.658, 36.068)
  line L1043 (93.5482, 23.5204) -> (93.5482, 24.4856)
  line L1044 (74.208, 36.068) -> (73.658, 36.068)
  line L1045 (42.46, 57.485) -> (42.46, 58.085)
  line L1046 (91.8718, 23.5204) -> (93.5482, 23.5204)
  line L1047 (73.408, 36.068) -> (72.858, 36.068)
  line L1048 (42.46, 58.085) -> (41.36, 58.085)
  line L1049 (73.025, 36.3728) -> (74.041, 36.3728)
  arc A485 (93.7122, 10.64) -> (93.7118, 10.64) centre (93.712, 10.64) ccw
  arc A486 (91.8348, 23.523) -> (91.8352, 23.523) centre (91.835, 23.523) ccw
  arc A487 (72.9832, 36.368) -> (72.9828, 36.368) centre (72.983, 36.368) ccw
  line L1050 (73.025, 36.3728) -> (74.041, 36.3728)
  line L1051 (73.408, 36.3728) -> (73.408, 35.7632)
  arc A488 (74.0828, 36.368) -> (74.0832, 36.368) centre (74.083, 36.368) ccw
  arc A489 (74.0832, 35.768) -> (74.0828, 35.768) centre (74.083, 35.768) ccw
  line L1052 (93.537, 9.71) -> (93.537, 10.61)
  line L1053 (93.537, 9.71) -> (93.537, 10.61)
  line L1054 (41.36, 58.085) -> (41.36, 57.485)
  line L1055 (73.658, 36.3728) -> (73.408, 36.3728)
  arc A490 (74.0832, 36.368) -> (74.0828, 36.368) centre (74.083, 36.368) ccw
  line L1056 (41.36, 57.485) -> (42.46, 57.485)
  line L1057 (73.658, 35.7632) -> (73.658, 36.3728)
  arc A491 (72.9828, 35.768) -> (72.9832, 35.768) centre (72.983, 35.768) ccw
  line L1058 (41.785, 58.0898) -> (41.785, 57.4802)
  line L1059 (74.083, 36.368) -> (72.983, 36.368)
  arc A492 (72.9832, 35.768) -> (72.9828, 35.768) centre (72.983, 35.768) ccw
  line L1060 (92.137, 9.71) -> (92.137, 10.61)
  line L1061 (74.041, 35.7632) -> (73.025, 35.7632)
  line L1062 (73.408, 36.068) -> (72.858, 36.068)
  line L1063 (93.537, 9.71) -> (93.537, 10.61)
  line L1064 (74.041, 36.3728) -> (74.041, 35.7632)
  arc A493 (74.0828, 35.768) -> (74.0832, 35.768) centre (74.083, 35.768) ccw
  line L1065 (72.983, 35.768) -> (74.083, 35.768)
  line L1066 (73.408, 35.7632) -> (73.658, 35.7632)
  line L1067 (94.696, 43.222) -> (94.696, 42.122)
  arc A494 (41.3598, 58.085) -> (41.3602, 58.085) centre (41.36, 58.085) ccw
  line L1068 (41.402, 58.0898) -> (42.418, 58.0898)
  line L1069 (41.785, 57.4802) -> (42.035, 57.4802)
  line L1070 (41.402, 57.4802) -> (41.402, 58.0898)
  arc A495 (72.9828, 36.368) -> (72.9832, 36.368) centre (72.983, 36.368) ccw
  line L1071 (42.035, 57.4802) -> (42.035, 58.0898)
  line L1072 (74.041, 36.3728) -> (74.041, 35.7632)
  line L1073 (41.235, 57.785) -> (41.785, 57.785)
  line L1074 (92.137, 9.71) -> (92.137, 10.61)
  line L1075 (73.408, 36.068) -> (72.858, 36.068)
  line L1076 (41.402, 58.0898) -> (42.418, 58.0898)
  line L1077 (74.041, 35.7632) -> (73.025, 35.7632)
  line L1078 (42.035, 57.785) -> (42.585, 57.785)
  line L1079 (42.418, 57.4802) -> (41.402, 57.4802)
  line L1080 (94.696, 42.122) -> (95.296, 42.122)
  arc A496 (94.696, 43.2222) -> (94.696, 43.2218) centre (94.696, 43.222) ccw
  line L1081 (94.6912, 43.18) -> (95.3008, 43.18)
  arc A497 (42.4598, 57.485) -> (42.4602, 57.485) centre (42.46, 57.485) ccw
  line L1082 (73.025, 35.7632) -> (73.025, 36.3728)
  line L1083 (41.235, 57.785) -> (41.785, 57.785)
  line L1084 (74.083, 35.768) -> (74.083, 36.368)
  line L1085 (74.208, 36.068) -> (73.658, 36.068)
  arc A498 (41.3598, 57.485) -> (41.3602, 57.485) centre (41.36, 57.485) ccw
  line L1086 (73.025, 35.7632) -> (73.025, 36.3728)
  line L1087 (72.983, 36.368) -> (72.983, 35.768)
  arc A499 (41.3602, 57.485) -> (41.3598, 57.485) centre (41.36, 57.485) ccw
  line L1088 (42.035, 57.785) -> (42.585, 57.785)
  arc A500 (94.696, 43.2218) -> (94.696, 43.2222) centre (94.696, 43.222) ccw
  line L1089 (95.3008, 43.18) -> (95.3008, 42.164)
  line L1090 (94.6912, 42.164) -> (94.6912, 43.18)
  line L1091 (42.418, 57.4802) -> (41.402, 57.4802)
  line L1092 (94.6912, 42.164) -> (94.6912, 43.18)
  arc A501 (42.4602, 57.485) -> (42.4598, 57.485) centre (42.46, 57.485) ccw
  arc A502 (94.696, 42.1222) -> (94.696, 42.1218) centre (94.696, 42.122) ccw
  line L1093 (95.3008, 42.164) -> (94.6912, 42.164)
  line L1094 (42.418, 58.0898) -> (42.418, 57.4802)
  line L1095 (94.6912, 43.18) -> (95.3008, 43.18)
  line L1096 (95.3008, 43.18) -> (95.3008, 42.164)
  arc A503 (41.3602, 58.085) -> (41.3598, 58.085) centre (41.36, 58.085) ccw
  line L1097 (42.035, 58.0898) -> (41.785, 58.0898)
  arc A504 (94.696, 42.1218) -> (94.696, 42.1222) centre (94.696, 42.122) ccw
  line L1098 (28.557, 21.1388) -> (29.573, 21.1388)
  line L1099 (34.297, 59.754) -> (33.197, 59.754)
  line L1100 (33.622, 57.422) -> (33.072, 57.422)
  arc A505 (6.35, 5.08) -> (6.35, 7.62) centre (6.35, 6.35) ccw
  line L1101 (33.197, 59.154) -> (34.297, 59.154)
  line L1102 (33.622, 57.422) -> (33.072, 57.422)
  line L1103 (28.515, 19.518) -> (29.615, 19.518)
  line L1104 (29.615, 21.134) -> (28.515, 21.134)
  line L1105 (33.622, 58.438) -> (33.072, 58.438)
  line L1106 (29.573, 20.1228) -> (29.573, 19.5132)
  line L1107 (28.557, 19.1068) -> (29.573, 19.1068)
  line L1108 (28.557, 18.4972) -> (28.557, 19.1068)
  line L1109 (28.515, 20.534) -> (29.615, 20.534)
  line L1110 (34.297, 58.738) -> (33.197, 58.738)
  arc A506 (33.1967, 58.738) -> (33.1972, 58.738) centre (33.197, 58.738) ccw
  arc A507 (34.2972, 58.138) -> (34.2967, 58.138) centre (34.297, 58.138) ccw
  line L1111 (29.19, 19.1068) -> (28.94, 19.1068)
  line L1112 (29.573, 18.4972) -> (28.557, 18.4972)
  line L1113 (33.622, 58.7428) -> (33.622, 58.1332)
  arc A508 (34.2972, 58.738) -> (34.2967, 58.738) centre (34.297, 58.738) ccw
  line L1114 (34.255, 58.1332) -> (33.239, 58.1332)
  line L1115 (33.197, 58.138) -> (34.297, 58.138)
  line L1116 (34.422, 58.438) -> (33.872, 58.438)
  arc A509 (33.1972, 58.738) -> (33.1967, 58.738) centre (33.197, 58.738) ccw
  line L1117 (33.872, 59.1492) -> (33.872, 59.7588)
  line L1118 (34.255, 58.7428) -> (34.255, 58.1332)
  line L1119 (33.197, 59.754) -> (33.197, 59.154)
  line L1120 (33.239, 58.1332) -> (33.239, 58.7428)
  line L1121 (33.622, 57.422) -> (33.072, 57.422)
  line L1122 (34.297, 59.154) -> (34.297, 59.754)
  line L1123 (33.872, 58.1332) -> (33.872, 58.7428)
  line L1124 (33.622, 58.438) -> (33.072, 58.438)
  line L1125 (34.255, 58.1332) -> (33.239, 58.1332)
  line L1126 (33.197, 58.738) -> (33.197, 58.138)
  line L1127 (34.297, 58.138) -> (34.297, 58.738)
  arc A510 (34.2967, 58.738) -> (34.2972, 58.738) centre (34.297, 58.738) ccw
  arc A511 (33.1972, 58.138) -> (33.1967, 58.138) centre (33.197, 58.138) ccw
  line L1128 (33.239, 58.7428) -> (34.255, 58.7428)
  line L1129 (83.693, 26.545) -> (83.693, 26.195)
  line L1130 (83.8708, 26.3398) -> (83.8708, 27.0002)
  arc A512 (83.843, 26.1633) -> (83.843, 26.2268) centre (83.843, 26.195) ccw
  line L1131 (83.543, 27.145) -> (83.543, 26.195)
  line L1132 (83.693, 26.545) -> (83.693, 26.195)
  line L1133 (77.0382, 47.115) -> (77.0382, 46.865)
  arc A513 (83.843, 26.2268) -> (83.843, 26.1633) centre (83.843, 26.195) ccw
  line L1134 (83.5152, 27.0002) -> (83.5152, 26.3398)
  line L1135 (77.0382, 46.865) -> (77.6478, 46.865)
  line L1136 (83.82, 29.3878) -> (83.82, 28.7782)
  arc A514 (83.7565, 28.7782) -> (83.8835, 28.7782) centre (83.82, 28.7782) ccw
  arc A515 (83.7565, 29.3878) -> (83.8835, 29.3878) centre (83.82, 29.3878) ccw
  line L1137 (82.804, 29.3878) -> (83.82, 29.3878)
  arc A516 (82.7405, 29.3878) -> (82.8675, 29.3878) centre (82.804, 29.3878) ccw
  arc A517 (82.8675, 28.7782) -> (82.7405, 28.7782) centre (82.804, 28.7782) ccw
  line L1138 (33.239, 56.1012) -> (33.239, 56.7108)
  line L1139 (33.872, 56.1012) -> (33.872, 56.7108)
  line L1140 (33.239, 56.7108) -> (34.255, 56.7108)
  line L1141 (34.255, 56.1012) -> (33.239, 56.1012)
  arc A518 (83.8622, 29.383) -> (83.8618, 29.383) centre (83.862, 29.383) ccw
  arc A519 (83.8835, 28.7782) -> (83.7565, 28.7782) centre (83.82, 28.7782) ccw
  arc A520 (33.3025, 56.1012) -> (33.1755, 56.1012) centre (33.239, 56.1012) ccw
  line L1142 (34.422, 56.406) -> (33.872, 56.406)
  line L1143 (33.622, 56.406) -> (33.072, 56.406)
  arc A521 (82.8675, 28.7782) -> (82.7405, 28.7782) centre (82.804, 28.7782) ccw
  line L1144 (33.872, 56.7108) -> (33.622, 56.7108)
  arc A522 (33.1755, 56.7108) -> (33.3025, 56.7108) centre (33.239, 56.7108) ccw
  line L1145 (33.622, 56.1012) -> (33.872, 56.1012)
  line L1146 (34.297, 56.706) -> (33.197, 56.706)
  arc A523 (82.7405, 28.7782) -> (82.8675, 28.7782) centre (82.804, 28.7782) ccw
  line L1147 (82.804, 28.7782) -> (82.804, 29.3878)
  arc A524 (82.8675, 29.3878) -> (82.7405, 29.3878) centre (82.804, 29.3878) ccw
  arc A525 (83.7565, 29.3878) -> (83.8835, 29.3878) centre (83.82, 29.3878) ccw
  arc A526 (82.7405, 29.3878) -> (82.8675, 29.3878) centre (82.804, 29.3878) ccw
  line L1148 (33.622, 56.406) -> (33.072, 56.406)
  line L1149 (83.187, 28.7782) -> (83.437, 28.7782)
  line L1150 (29.615, 20.534) -> (29.615, 21.134)
  arc A527 (33.3025, 56.7108) -> (33.1755, 56.7108) centre (33.239, 56.7108) ccw
  arc A528 (82.7618, 28.783) -> (82.7622, 28.783) centre (82.762, 28.783) ccw
  line L1151 (83.862, 29.383) -> (82.762, 29.383)
  arc A529 (83.8835, 29.3878) -> (83.7565, 29.3878) centre (83.82, 29.3878) ccw
  line L1152 (83.437, 28.7782) -> (83.437, 29.3878)
  arc A530 (83.8835, 28.7782) -> (83.7565, 28.7782) centre (83.82, 28.7782) ccw
  line L1153 (34.255, 56.7108) -> (34.255, 56.1012)
  line L1154 (83.187, 29.3878) -> (83.187, 28.7782)
  arc A531 (82.7405, 28.7782) -> (82.8675, 28.7782) centre (82.804, 28.7782) ccw
  arc A532 (34.2967, 56.106) -> (34.2972, 56.106) centre (34.297, 56.106) ccw
  arc A533 (82.8675, 29.3878) -> (82.7405, 29.3878) centre (82.804, 29.3878) ccw
  arc A534 (33.1972, 56.706) -> (33.1967, 56.706) centre (33.197, 56.706) ccw
  line L1155 (34.255, 56.1012) -> (33.239, 56.1012)
  arc A535 (33.1755, 56.7108) -> (33.3025, 56.7108) centre (33.239, 56.7108) ccw
  line L1156 (33.622, 56.7108) -> (33.622, 56.1012)
  arc A536 (33.1967, 56.706) -> (33.1972, 56.706) centre (33.197, 56.706) ccw
  arc A537 (34.2972, 56.106) -> (34.2967, 56.106) centre (34.297, 56.106) ccw
  arc A538 (82.7622, 28.783) -> (82.7618, 28.783) centre (82.762, 28.783) ccw
  arc A539 (33.3025, 56.1012) -> (33.1755, 56.1012) centre (33.239, 56.1012) ccw
  arc A540 (83.8618, 28.783) -> (83.8622, 28.783) centre (83.862, 28.783) ccw
  line L1157 (83.82, 29.3878) -> (83.82, 28.7782)
  line L1158 (82.804, 28.7782) -> (82.804, 29.3878)
  line L1159 (20.576, 32.385) -> (20.026, 32.385)
  arc A541 (33.1972, 56.106) -> (33.1967, 56.106) centre (33.197, 56.106) ccw
  arc A542 (34.3185, 56.7108) -> (34.1915, 56.7108) centre (34.255, 56.7108) ccw
  line L1160 (83.82, 28.7782) -> (82.804, 28.7782)
  arc A543 (82.7618, 29.383) -> (82.7622, 29.383) centre (82.762, 29.383) ccw
  line L1161 (82.762, 28.783) -> (83.862, 28.783)
  line L1162 (82.804, 29.3878) -> (83.82, 29.3878)
  line L1163 (83.437, 29.3878) -> (83.187, 29.3878)
  line L1164 (83.82, 28.7782) -> (82.804, 28.7782)
  line L1165 (20.576, 32.385) -> (20.026, 32.385)
  arc A544 (34.1915, 56.7108) -> (34.3185, 56.7108) centre (34.255, 56.7108) ccw
  arc A545 (33.3025, 56.7108) -> (33.1755, 56.7108) centre (33.239, 56.7108) ccw
  arc A546 (34.1915, 56.7108) -> (34.3185, 56.7108) centre (34.255, 56.7108) ccw
  arc A547 (83.8618, 29.383) -> (83.8622, 29.383) centre (83.862, 29.383) ccw
  arc A548 (82.7622, 29.383) -> (82.7618, 29.383) centre (82.762, 29.383) ccw
  line L1166 (33.622, 56.406) -> (33.072, 56.406)
  line L1167 (82.762, 29.383) -> (82.762, 28.783)
  line L1168 (83.437, 29.083) -> (83.987, 29.083)
  line L1169 (83.437, 29.083) -> (83.987, 29.083)
  arc A549 (34.2972, 57.122) -> (34.2967, 57.122) centre (34.297, 57.122) ccw
  arc A550 (34.2967, 57.122) -> (34.2972, 57.122) centre (34.297, 57.122) ccw
  line L1170 (82.637, 29.083) -> (83.187, 29.083)
  arc A551 (83.8835, 29.3878) -> (83.7565, 29.3878) centre (83.82, 29.3878) ccw
  arc A552 (83.7565, 28.7782) -> (83.8835, 28.7782) centre (83.82, 28.7782) ccw
  arc A553 (83.8622, 28.783) -> (83.8618, 28.783) centre (83.862, 28.783) ccw
  arc A554 (34.2972, 57.722) -> (34.2967, 57.722) centre (34.297, 57.722) ccw
  line L1171 (33.197, 57.122) -> (34.297, 57.122)
  line L1172 (33.622, 57.7268) -> (33.622, 57.1172)
  line L1173 (83.862, 28.783) -> (83.862, 29.383)
  arc A555 (6.35, 5.08) -> (6.35, 7.62) centre (6.35, 6.35) ccw